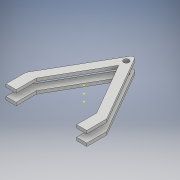
# Autodesk Inventor part: tri
Saved by Autodesk Inventor 2018 (Build 220112000, 112)
## iProperties
Created: 2021-12-08
Part Number: tri
Material: Generic
Document SubType Name: Modeling
Designer: cs1190490
Density: 1 g/cm^3
Appearance: Default
Author: cs1190490
Autodesk Inventor part; units mm, degrees
ref_plane "XZ Plane" through (0, 0, 0) normal (0, 1, 0) x (-1, 0, 0)
sketch "Sketch5" plane through (0, 0, 0) normal (0, 0, 1) x (1, 0, 0)
  line L0 (0, 299.9912) -> (259.8, -149.9956)
  line L1 (259.8, -149.9956) -> (-259.8, -149.9956)
  line L2 (-259.8, -149.9956) -> (0, 299.9912)
  point P0 (0, 0)
  point P1 (0, 0)
  dimension "d12" = 519.6
  constraints: 6 end point, 1 coincident, 7 other
  measures "d12" distance of L0.start L0.end
extrude "Extrusion5" add sketch "Sketch5" along normal blind 17.5
sketch "Sketch6" plane through (0, 0, 17.5) normal (0, 0, 1) x (1, 0, 0)
  point P0 (0, 0)
sketch "Sketch7" plane through (0, 0, 17.5) normal (0, 0, 1) x (1, 0, 0)
  point P0 (0, 0)
sketch "Sketch8" plane through (0, 0, 17.5) normal (0, 0, 1) x (1, 0, 0)
  line L0 (0, 199.9912) -> (173.1975, -99.9956)
  line L1 (173.1975, -99.9956) -> (-173.1975, -99.9956)
  line L2 (-173.1975, -99.9956) -> (0, 199.9912)
  line L3 (259.8, -149.9956) -> (0, 299.9912) projected
  point P0 (0, 0)
  point P1 (0, 0)
  dimension "d15" = 50
  constraints: 6 end point, 1 coincident, 7 other
  measures "d15" distance between parallel lines of L0 L3
extrude "Extrusion6" cut sketch "Sketch8" against normal blind 323.25
sketch "Sketch9" plane through (0, 0, 17.5) normal (0, 0, 1) x (1, 0, 0)
  line L0 (-297.8185, -99.9956) -> (278.7912, -99.9956)
  line L1 (278.7912, -99.9956) -> (278.7912, -149.9956)
  line L2 (278.7912, -149.9956) -> (-297.8185, -149.9956)
  line L3 (-297.8185, -149.9956) -> (-297.8185, -99.9956)
  point P0 (0, 0)
  constraints: 8 end point, 2 parallel, 1 horizontal, 1 perpendicular
extrude "Extrusion7" cut sketch "Sketch9" against normal blind 130.25
ref_plane "Work Plane2" through (0, 0, -22.5) normal (0, 0, -1) x (-1, 0, 0)
sketch "Sketch10" plane through (0, 0, -22.5) normal (0, 0, -1) x (-1, 0, 0)
  point P0 (0, 0)
mirror "Mirror3" about plane through (0, 0, -22.5) normal (0, 0, -1) of "Extrusion5", "Extrusion6", "Extrusion7"
fillet "Fillet3" radius 15 2 edges at (0, 299.9912, -53.75) (0, 299.9912, 8.75)
sketch "Sketch11" plane through (230.9325, -99.9956, -62.5) normal (0, 0, -1) x (-1, 0, 0)
  circle A0 centre (230.9325, 343.0479) radius 15.366
  point P0 (230.9325, 99.9956)
  constraints: 1 centre point
extrude "Extrusion8" cut sketch "Sketch11" against normal blind 474.75
sketch "Sketch12" plane through (230.9325, -99.9956, -62.5) normal (0, 0, -1) x (-1, 0, 0)
  line L0 (461.865, 0) -> (243.9229, 377.4868) projected
  line L1 (461.865, 0) -> (462.5144, -114.8)
  line L2 (404.1299, 0) -> (230.9325, 299.9868) projected
  line L3 (404.1299, 0) -> (404.1299, -114.8)
  line L4 (57.735, 0) -> (57.735, -112.3529)
  line L5 (57.735, 0) -> (0, 0) projected
  line L6 (0, 0) -> (0, -112.3529)
  line L7 (0, -112.3529) -> (57.735, -112.3529)
  line L8 (462.5144, -114.8) -> (404.1299, -114.8)
  line L9 (461.865, 0) -> (404.1299, 0)
  line L10 (0, 0) -> (57.735, 0) projected
  line L11 (57.735, 0) -> (0, 0)
  point P0 (230.9325, 99.9956)
  dimension "d24" = 114.8
  constraints: 16 end point, 2 vertical, 1 collinear, 1 horizontal, 1 parallel, 1 perpendicular, 1 point on line
  measures "d24" vertical distance of L1.start L1.end
extrude "Extrusion9" add sketch "Sketch12" against normal blind 17.5 contours L1 L8 L3 L9
sketch "Sketch13" plane through (230.9325, -99.9956, -62.5) normal (0, 0, -1) x (-1, 0, 0)
  point P0 (230.9325, 99.9956)
ref_plane "Work Plane3" through (0, 0, -22.5) normal (1, 0, 0) x (0, 1, 0)
mirror "Mirror4" about plane through (0, 0, -22.5) normal (1, 0, 0) of "Extrusion9"
mirror "Mirror5" about plane through (0, 0, -22.5) normal (0, 0, -1) of "Extrusion9", "Mirror4"
ref_plane "Work Plane4" through (0, 0, -22.5) normal (0, 0, -1) x (-1, 0, 0)
body "Solid2"
